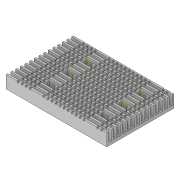
# Autodesk Inventor part: 6089-104-RevA_HEATSINK_KU15P
Saved by Autodesk Inventor 2017.3 (Build 213256000, 256)
## iProperties
Created: 2019-01-23
Part Number: 6089-104-RevA_HEATSINK_KU15P
Material: Generic
Document SubType Name: Modeling
Designer: crs5
Density: 1 g/cm^3
Appearance: Default
Author: crs5
Autodesk Inventor part; units mm, degrees
ref_plane "YZ Plane" through (0, 0, 0) normal (1, 0, 0) x (0, 1, 0)
ref_plane "XZ Plane" through (0, 0, 0) normal (0, 1, 0) x (-1, 0, 0)
ref_plane "XY Plane" through (0, 0, 0) normal (0, 0, 1) x (1, 0, 0)
sketch "Sketch1" plane through (0, 0, 0) normal (0, 1, 0) x (-1, 0, 0)
  line L0 (0, 0) -> (125, 0)
  line L1 (125, 0) -> (125, -83.5)
  line L2 (125, -83.5) -> (0, -83.5)
  line L3 (0, -83.5) -> (0, 0)
  dimension "d0" = 83.5
  dimension "d1" = 125
  constraints: 8 end point, 2 parallel, 1 horizontal, 1 perpendicular
  measures "d0" distance of L2.end L0.start
  measures "d1" distance of L0.start L0.end
extrude "Extrusion1" add sketch "Sketch1" along normal blind 15.4
hole "Hole1" at (-20, 15.4, -18.5214) direction (0, -1, 0) diameter 6 end through all counterbore diameter 8.9 counterbore depth 13.5
pattern_linear "Rectangular Pattern1" count 3 spacing 23.2286 along (0, 0, -1) count 2 spacing 67 along (-1, 0, 0) of "Hole1"
hole "Hole2" at (-53.5, 15.4, -41.75) direction (0, -1, 0) diameter 1.8 end through all
sketch "Sketch2" plane through (0, 0, 0) normal (1, 0, 0) x (0, 0, -1)
  line L0 (0, 15.4) -> (83.5, 15.4) projected
  line L1 (2.2, 15.4) -> (5.8071, 15.4)
  line L2 (5.8071, 15.4) -> (5.8071, 4)
  line L3 (5.8071, 4) -> (2.2, 4)
  line L4 (2.2, 4) -> (2.2, 15.4)
  line L5 (83.5, 0) -> (0, 0) projected
  line L6 (0, 0) -> (0, 15.4) projected
  dimension "d28" = 4
  dimension "d29" = 2.2
  dimension "d30" = 3.6071
  constraints: 8 end point, 2 parallel, 1 horizontal, 1 perpendicular, 1 point on line
  measures "d28" distance between parallel lines of L5 L3
  measures "d29" distance between parallel lines of L6 L4
  measures "d30" distance of L2.end L3.end
extrude "Extrusion2" cut sketch "Sketch2" against normal up to next
pattern_linear "Rectangular Pattern2" count 14 spacing 5.8071 along (0, 0, -1) of "Extrusion2"
sketch "Sketch3" plane through (-125, 0, 0) normal (0, 0, 1) x (1, 0, 0)
  line L0 (42.3119, 15.4) -> (100.6881, 15.4) projected
  line L1 (95.8, 15.4) -> (97.3, 15.4)
  line L2 (97.3, 15.4) -> (97.3, 13.9)
  line L3 (97.3, 13.9) -> (95.8, 13.9)
  line L4 (95.8, 13.9) -> (95.8, 15.4)
  line L5 (125, 0) -> (125, 15.4) projected
  dimension "d36" = 1.5
  dimension "d37" = 1.5
  dimension "d38" = 27.7
  constraints: 8 end point, 2 parallel, 1 horizontal, 1 perpendicular, 1 point on line
  measures "d36" distance of L2.end L3.end
  measures "d37" distance of L1.end L2.end
  measures "d38" distance between parallel lines of L5 L2
extrude "Extrusion3" cut sketch "Sketch3" against normal blind 83.5
pattern_linear "Rectangular Pattern3" count 11 spacing 5 along (-1, 0, 0) of "Extrusion3"
sketch "Sketch5" plane through (-125, 0, 0) normal (0, 0, 1) x (1, 0, 0)
  line L0 (97.3, 15.4) -> (125, 15.4) projected
  line L1 (112.7, 15.4) -> (114.2, 15.4)
  line L2 (114.2, 15.4) -> (114.2, 13.9)
  line L3 (114.2, 13.9) -> (112.7, 13.9)
  line L4 (112.7, 13.9) -> (112.7, 15.4)
  line L5 (125, 0) -> (125, 15.4) projected
  dimension "d45" = 1.5
  dimension "d46" = 1.5
  dimension "d47" = 12.3
  constraints: 8 end point, 2 parallel, 1 horizontal, 1 perpendicular, 1 point on line
  measures "d45" distance of L1.end L2.end
  measures "d46" distance of L2.end L3.end
  measures "d47" distance between parallel lines of L5 L4
extrude "Extrusion4" cut sketch "Sketch5" against normal blind 83.5
pattern_linear "Rectangular Pattern4" count 2 spacing 5 along (1, 0, 0) of "Extrusion4"
sketch "Sketch6" plane through (-125, 0, 0) normal (0, 0, 1) x (1, 0, 0)
  line L0 (0, 15.4) -> (33.6881, 15.4) projected
  line L1 (28.8, 15.4) -> (30.3, 15.4)
  line L2 (30.3, 15.4) -> (30.3, 13.9)
  line L3 (30.3, 13.9) -> (28.8, 13.9)
  line L4 (28.8, 13.9) -> (28.8, 15.4)
  line L5 (125, 0) -> (125, 15.4) projected
  dimension "d53" = 1.5
  dimension "d54" = 1.5
  dimension "d55" = 94.7
  constraints: 8 end point, 2 parallel, 1 horizontal, 1 perpendicular, 1 point on line
  measures "d53" distance of L2.end L3.end
  measures "d54" distance of L1.end L2.end
  measures "d55" distance between parallel lines of L5 L2
extrude "Extrusion5" cut sketch "Sketch6" against normal blind 83.5
pattern_linear "Rectangular Pattern5" count 4 spacing 5 along (-1, 0, 0) of "Extrusion5"
equation "\"d0\" = hs_width"
equation "\"d1\" = hs_length_KU15P"
equation "\"d6\" = hole_dia"
equation "\"d4\" = hole_ll_x"
equation "\"d5\" = hole_ll_y"
equation "\"d8\" = spring_hole_ID"
equation "\"d9\" = spring_hole_total_depth"
equation "\"d15\" = hole_lc_x - hole_ll_x"
equation "\"d18\" = hole_ul_y - hole_ll_y"
equation "\"d19\" = hole_fpga_center_x"
equation "\"d20\" = hole_fpga_center_y"
equation "\"d23\" = spring_hole_ID"
equation "\"d24\" = spring_hole_total_depth"
equation "\"d28\" = hs_base_thickness"
equation "\"d29\" = hs_fin_thickness"
equation "\"d30\" = hs_fin_gap"
equation "\"d31\" = hs_overall_height"
equation "\"d35\" = hs_pitch"
equation "\"d39\" = hs_width"
equation "\"d48\" = hs_width"
equation "\"d56\" = hs_width"
equation "\"hs_length_KU15P\" = 125"
equation "\"hs_width\" = 83.5"
equation "\"hs_base_thickness\" = 4"
equation "\"hs_overall_height\" = 15"
equation "\"hs_fin_thickness\" = 2.2"
equation "\"hole_y_spacing\" = 67"
equation "\"hole_dia\" = 6"
equation "\"spring_OD\" = 7.9"
equation "\"spring_free_length\" = 9.7"
equation "\"spring_compressed_length\" = 4.8"
equation "\"spring_OD_clearance\" = 1"
equation "\"spring_insertion_depth\" = 2.5"
equation "\"hs_fin_gap\" = 3.60714"
equation "\"hs_pitch\" = 5.80714"
equation "\"hs_center_offset\" = 0"
equation "\"hole_x_spacing\" = 23.22857"
equation "\"hole_ll_x\" = 18.52143"
equation "\"hole_ll_y\" = 20"
equation "\"hole_lc_x\" = 41.75"
equation "\"hole_lr_x\" = 64.97857"
equation "\"hole_ul_x\" = 18.52143"
equation "\"hole_ul_y\" = 87"
equation "\"hole_uc_x\" = 41.75"
equation "\"hole_uc_y\" = 87"
equation "\"hole_ur_x\" = 64.97857"
equation "\"hole_ur_y\" = 87"
equation "\"hole_fpga_center_x\" = 41.75"
equation "\"hole_fpga_center_y\" = 53.5"
equation "\"spring_hole_ID\" = 8.9"
equation "\"spring_hole_total_depth\" = 13.5"
body "Solid1"
